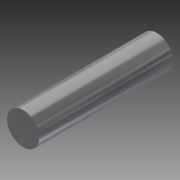
# Autodesk Inventor part: panGearShaft1
Saved by Autodesk Inventor 2013 (Build 170138000, 138)
## iProperties
Created: 2014-06-30
Part Number: panGearShaft1
Material: Stainless Steel
Document SubType Name: Modeling
Designer: Nano
Density: 8.08 g/cm^3
Mass: 6.75952 g
Surface Area: 5.90314 cm^2
Volume: 0.836574 cm^3
Author: Nano
Autodesk Inventor part; units mm, degrees
ref_plane "YZ Plane" through (0, 0, 0) normal (1, 0, 0) x (0, 1, 0)
ref_plane "XZ Plane" through (0, 0, 0) normal (0, 1, 0) x (-1, 0, 0)
ref_plane "XY Plane" through (0, 0, 0) normal (0, 0, 1) x (1, 0, 0)
ref_plane "Work Plane1" through (0, 0, 0) normal (0, 0, 1) x (1, 0, 0)
sketch "Sketch1" plane through (0, 0, 0) normal (0, 0, 1) x (1, 0, 0)
  circle A0 centre (0, 25.4) radius 3.175 projected
  point P0 (0, 0)
ref_plane "Work Plane2" through (-93.3376, -133.5722, -26.416) normal (0, 0, -1) x (0, 1, 0)
extrude "Extrusion1" add sketch "Sketch1" against normal up to surface (26.416 mm away)
body "Solid1"
